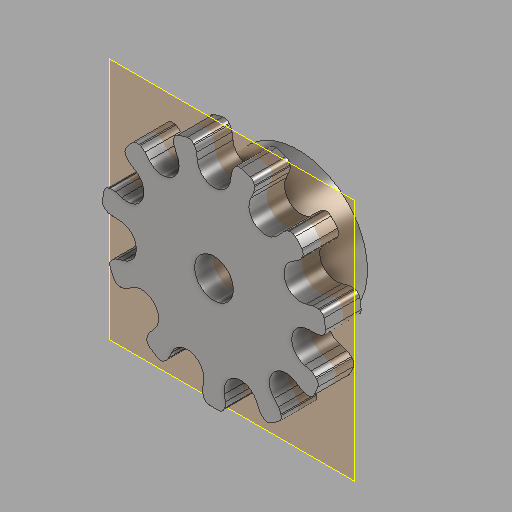
# Autodesk Inventor part: Piñon Motriz
Saved by Autodesk Inventor 2024.3 (Build 283343010, 343A)
## iProperties
Created: 2025-05-17
Part Number: Piñon Motriz
Material: Steel, Galvanized
Document SubType Name: Modeling
Designer: Gary
Density: 7.85 g/cm^3
Appearance: Galvanized
Author: Gary
Autodesk Inventor part; units mm, degrees
ref_plane "YZ Plane" through (0, 0, 0) normal (1, 0, 0) x (0, 1, 0)
ref_plane "XZ Plane" through (0, 0, 0) normal (0, 1, 0) x (-1, 0, 0)
ref_plane "XY Plane" through (0, 0, 0) normal (0, 0, 1) x (1, 0, 0)
sketch "Sketch1" plane through (0, 0, 0) normal (0, 0, 1) x (1, 0, 0)
  circle A0 centre (0, 0) radius 78.885
  circle A1 centre (0, 0) radius 16
  circle A2 centre (0, 0) radius 92.698
  circle A3 centre (0, 78.885) radius 13.813
  circle A4 centre (-42.6485, 66.3623) radius 13.813
  circle A5 centre (-71.7563, 32.77) radius 13.813
  circle A6 centre (-78.0821, -11.2265) radius 13.813
  circle A7 centre (-59.6173, -51.6587) radius 13.813
  circle A8 centre (-22.2245, -75.6896) radius 13.813
  circle A9 centre (22.2245, -75.6896) radius 13.813
  circle A10 centre (59.6173, -51.6587) radius 13.813
  circle A11 centre (78.0821, -11.2265) radius 13.813
  circle A12 centre (71.7563, 32.77) radius 13.813
  circle A13 centre (42.6485, 66.3623) radius 13.813
  circle A14 centre (0, 0) radius 65.072
  line L0 (13.76, 77.6757) -> (15.0303, 85.4062)
  line L1 (30.419, 72.7841) -> (33.5973, 79.9243)
  line L2 (15.0303, 85.4062) -> (18.9701, 90.7362)
  line L3 (33.1803, 86.5563) -> (33.5973, 79.9243)
  line L4 (-33.5297, 79.9743) -> (-33.097, 86.5881)
  line L5 (-30.419, 72.7841) -> (-33.5297, 79.9743)
  line L6 (-18.8828, 90.7544) -> (-14.9465, 85.4006)
  line L7 (-13.76, 77.6757) -> (-14.9465, 85.4006)
  line L8 (-71.4444, 49.1511) -> (-74.6561, 54.949)
  line L9 (-64.9402, 44.7841) -> (-71.4444, 49.1511)
  line L10 (-64.9507, 66.1387) -> (-58.7448, 63.7629)
  line L11 (-53.5702, 57.9057) -> (-58.7448, 63.7629)
  line L12 (-86.6759, 2.7228) -> (-92.5123, 5.8639)
  line L13 (-78.8433, 2.5655) -> (-86.6759, 2.7228)
  line L14 (-90.3973, 20.5244) -> (-83.8921, 21.8809)
  line L15 (-76.3724, 19.7511) -> (-83.8921, 21.8809)
  line L16 (-74.3885, -44.57) -> (-80.9966, -45.0829)
  line L17 (-67.7142, -40.4677) -> (-74.3885, -44.57)
  line L18 (-87.1433, -31.6063) -> (-82.4043, -26.9481)
  line L19 (-74.9268, -24.6743) -> (-82.4043, -26.9481)
  line L20 (-38.4832, -77.7121) -> (-43.765, -81.7162)
  line L21 (-35.0863, -70.6526) -> (-38.4832, -77.7121)
  line L22 (-56.222, -73.7021) -> (-54.7536, -67.2213)
  line L23 (-49.6925, -61.2658) -> (-54.7536, -67.2213)
  line L24 (9.6402, -86.1812) -> (7.3617, -92.4052)
  line L25 (8.6812, -78.4059) -> (9.6402, -86.1812)
  line L26 (-7.4506, -92.3981) -> (-9.7191, -86.1522)
  line L27 (-8.6812, -78.4059) -> (-9.7191, -86.1522)
  line L28 (54.7029, -67.2883) -> (56.1511, -73.7562)
  line L29 (49.6925, -61.2658) -> (54.7029, -67.2883)
  line L30 (43.6864, -81.7583) -> (38.4012, -77.7304)
  line L31 (35.0863, -70.6526) -> (38.4012, -77.7304)
  line L32 (82.3979, -27.0319) -> (87.1129, -31.6901)
  line L33 (74.9268, -24.6743) -> (82.3979, -27.0319)
  line L34 (80.9532, -45.1608) -> (74.3293, -44.6297)
  line L35 (67.7142, -40.4677) -> (74.3293, -44.6297)
  line L36 (83.932, 21.8069) -> (90.417, 20.4374)
  line L37 (76.3724, 19.7511) -> (83.932, 21.8069)
  line L38 (92.5179, 5.7749) -> (86.6585, 2.6406)
  line L39 (78.8433, 2.5655) -> (86.6585, 2.6406)
  line L40 (58.8184, 63.7223) -> (65.0143, 66.0761)
  line L41 (53.5702, 57.9057) -> (58.8184, 63.7223)
  line L42 (74.7089, 54.8771) -> (71.4742, 49.0725)
  line L43 (64.9402, 44.7841) -> (71.4742, 49.0725)
  point P0 (-53.5702, 57.9057)
  point P1 (-64.9402, 44.7841)
  point P2 (-76.3724, 19.7511)
  point P3 (-78.8433, 2.5655)
  point P4 (-74.9268, -24.6743)
  point P5 (-67.7142, -40.4677)
  point P6 (-49.6925, -61.2658)
  point P7 (-8.6812, -78.4059)
  point P8 (8.6812, -78.4059)
  point P9 (35.0863, -70.6526)
  point P10 (49.6925, -61.2658)
  point P11 (67.7142, -40.4677)
  point P12 (74.9268, -24.6743)
  point P13 (78.8433, 2.5655)
  point P14 (76.3724, 19.7511)
  point P15 (64.9402, 44.7841)
  point P16 (53.5702, 57.9057)
  point P17 (-13.76, 77.6757)
  dimension "d0" = 157.77
  dimension "d1" = 32
  dimension "d2" = 185.396
  dimension "d5" = 360
  dimension "d9" = 360
  constraints: 88 end point, 13 centre point, 5 point on circle, 4 coincident, 141 other
  measures "d0" diameter of A0
  measures "d1" diameter of A1
  measures "d2" diameter of A2
extrude "Extrusion1" add sketch "Sketch1" along normal blind 29.44 contours A11 A14 A12 A0 | A0 L37 L36 A2 L38 L39 | L33 L32 A2 L34 L35 A0 | A0 A10 A14 A11 | A14 | A12 A14 A13 A0 | A0 L41 L40 A2 L42 L43 | A10 A0 A9 A14 | L29 L28 A2 L30 L31 A0 | A14 A3 A0 A13 | A9 A0 A8 A14 | A0 L0 L2 A2 L3 L1 | A14 A4 A0 A3 | L25 L24 A2 L26 L27 A0 | A8 A0 A7 A14 | A0 L5 L4 A2 L6 L7 | A14 A5 A0 A4 | L21 L20 A2 L22 L23 A0 | A7 A0 A6 A14 | A0 L9 L8 A2 L10 L11 | A14 A6 A0 A5 | L17 L16 A2 L18 L19 A0 | A0 L13 L12 A2 L14 L15
sketch "Sketch2" plane through (0, 0, 0) normal (0, 0, -1) x (-1, 0, 0)
  circle A0 centre (0, 0) radius 16 projected
  circle A1 centre (0, 0) radius 57.5
  dimension "d13" = 115
  constraints: 1 centre point, 1 coincident
  measures "d13" diameter of A1
extrude "Extrusion2" add sketch "Sketch2" along normal blind 40
fillet "Fillet1" radius 5 1 edges at (-64.9507, 66.1387, 14.72)
fillet "Fillet2" radius 5 1 edges at (-74.6561, 54.949, 14.72)
pattern_circular "Circular Pattern1" count 11 over 360 about axis through (0, 0, 0) along (0, 0, 1) of "Fillet2", "Fillet1"
fillet "Fillet3" radius 10 1 edges at (-38.4832, -77.7121, 14.72)
fillet "Fillet4" radius 10 1 edges at (-54.7536, -67.2213, 14.72)
pattern_circular "Circular Pattern2" count 11 over 360 about axis through (0, 0, 0) along (0, 0, 1) of "Fillet4", "Fillet3"
ref_plane "Work Plane1" through (0, 0, 14.72) normal (0, 0, 1) x (1, 0, 0)
body "Solid1"
